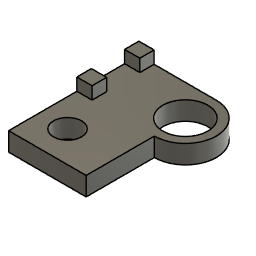
armservo v4 (Autodesk Fusion 360 design; units mm, degrees)
Autodesk Fusion 360 part; units mm, degrees
sketch "Esquisse1" plane through (0, 0, 0) normal (0, 1, 0) x (1, 0, 0)
  circle A0 centre (0, 0) radius 36.2394
  line L0 (-100, 50) -> (-125, 50)
  line L1 (-125, 50) -> (-125, -49.0109)
  circle A1 centre (0, 0) radius 50
  line L2 (-125, 50) -> (0, 50)
  line L3 (0, -50) -> (-125, -50)
  line L4 (-125, -50) -> (-125, 50)
  line L5 (-100, -50) -> (-100, -26.5854)
  line L6 (-100, -26.5854) -> (-124.9543, -26.5854)
  line L7 (-100, 50) -> (-100, 27)
  line L8 (-100, 27) -> (-125, 27)
  point P0 (-100, -50)
  point P1 (-100, -26.5854)
  point P2 (-100, 0)
  point P3 (-100, 27)
  point P4 (-100, 50)
  dimension "d3" = 100
  constraint horizontal L0
  constraint vertical L1
  constraint concentric A0 A1
  constraint horizontal L2
  constraint horizontal L3
  constraint vertical L4
  constraint coincident A1 L3.start
  constraint coincident L3 P0
  constraint coincident L0.start L7.start
  constraint coincident P0 L5.start
  constraint coincident P1 L5.end
  constraint perpendicular L3 L5
  constraint perpendicular L1 L6
  constraint coincident P4 L0.start
  constraint coincident P3 L7.end
  constraint perpendicular L2 L7
  constraint perpendicular L1 L8
  constraint coincident A1 L2.end
  constraint tangent A1 L2
  measures "d3" diameter of A1
extrude "Extrusion1" add sketch "Esquisse1" along normal blind 20 contours A1
sketch "Esquisse2" plane through (0, 20, 0) normal (0, 1, 0) x (-1, 0, 0)
  circle A0 centre (0, 0) radius 36.2394
  circle A1 centre (0, 0) radius 50
extrude "Extrusion3" add sketch "Esquisse1" along normal blind 20 contours L0 L1 L2 L4 L7 L8 | L1 A1 L2 L3 L4 L7 L8
sketch "Esquisse3" plane through (0, 20, 0) normal (0, 1, 0) x (-1, 0, 0)
  circle A0 centre (0, 0) radius 36.2394
  arc A1 (0, 50) -> (0, -50) centre (0, 0) ccw
  line L0 (0, -50) -> (125, -50)
  line L1 (125, -50) -> (125, 50)
  line L2 (125, 50) -> (0, 50)
  line L3 (125, -50) -> (100.4173, -50)
  line L4 (100.4173, -50) -> (100.4173, -26.9813)
  line L5 (100.4173, -26.9813) -> (125, -26.9813)
  line L6 (125, -26.9813) -> (125, -50)
  line L7 (125, 50) -> (100.4173, 50)
  line L8 (100.4173, 50) -> (100.4173, 26.5121)
  line L9 (100.4173, 26.5121) -> (125, 26.5121)
  line L10 (125, 26.5121) -> (125, 50)
  constraint horizontal L3
  constraint vertical L4
  constraint horizontal L5
  constraint vertical L6
  constraint coincident L0.end L1.start
  constraint horizontal L7
  constraint vertical L8
  constraint horizontal L9
  constraint vertical L10
  constraint coincident L1.end L2.start
extrude "Extrusion4" add sketch "Esquisse3" along normal blind 30 contours L1 L2 L7 L8 L9 L10 | L0 L1 L3 L4 L5 L6
sketch "Esquisse4" plane through (0, 0, 50) normal (0, 0, 1) x (1, 0, 0)
  line L0 (-125, 0) -> (0, 0)
  line L1 (0, 0) -> (0, 20)
  line L2 (0, 20) -> (-100.4173, 20)
  line L3 (-100.4173, 20) -> (-100.4173, 50)
  line L4 (-100.4173, 50) -> (-125, 50)
  line L5 (-125, 50) -> (-125, 0)
  line L6 (0, 0) -> (-125, 0)
  line L7 (-125, 0) -> (-125, 20)
  line L8 (-125, 20) -> (0, 20)
  line L9 (0, 20) -> (0, 0)
  constraint horizontal L6
  constraint vertical L7
  constraint horizontal L8
  constraint vertical L9
  constraint coincident L5 L7.end
  constraint coincident L0.end L1.start
extrude "Extrusion5" add sketch "Esquisse4" along normal blind 110 contours L0 L1 L2 L5 L6 L7 L8 L9
sketch "Esquisse5" plane through (0, 20, 0) normal (0, 1, 0) x (-1, 0, 0)
  line L0 (100.4173, 26.5121) -> (100.4173, 50)
  line L1 (100.4173, 50) -> (125, 50)
  line L2 (125, 50) -> (125, 160)
  line L3 (125, 160) -> (0, 160)
  line L4 (0, 160) -> (0, 50)
  arc A0 (0, 50) -> (0, -50) centre (0, 0) ccw
  line L5 (0, -50) -> (100.4173, -50)
  line L6 (100.4173, -50) -> (100.4173, -26.9813)
  line L7 (100.4173, -26.9813) -> (125, -26.9813)
  line L8 (125, -26.9813) -> (125, 26.5121)
  line L9 (125, 26.5121) -> (100.4173, 26.5121)
  circle A1 centre (0, 0) radius 36.2394
  circle A2 centre (80, 110) radius 25
  dimension "d14" = 50
  measures "d14" diameter of A2
extrude "Extrusion6" cut sketch "Esquisse5" against normal blind 20 contours A2
extrude "Extrusion7" cut 2 faces at (-108.6116, 50, -34.6542) (-108.6116, 50, 42.1707) along direction (0, -1, 0) blind 10
extrude "Extrusion8" add 1 faces at (-73.7992, 0, 13.676) along direction (0, -1, 0) blind 10
sketch "Esquisse6" plane through (0, 20, 0) normal (0, 1, 0) x (-1, 0, 0)
  circle A0 centre (80, 110) radius 25
  line L0 (100.4173, 26.5121) -> (100.4173, 50)
  line L1 (100.4173, 50) -> (125, 50)
  line L2 (125, 50) -> (125, 160)
  line L3 (125, 160) -> (0, 160)
  line L4 (0, 160) -> (0, 50)
  arc A1 (0, 50) -> (0, -50) centre (0, 0) ccw
  line L5 (0, -50) -> (100.4173, -50)
  line L6 (100.4173, -50) -> (100.4173, -26.9813)
  line L7 (100.4173, -26.9813) -> (125, -26.9813)
  line L8 (125, -26.9813) -> (125, 26.5121)
  line L9 (125, 26.5121) -> (100.4173, 26.5121)
  circle A2 centre (0, 0) radius 36.2394
  circle A3 centre (80, 110) radius 22.5
  dimension "d21" = 45
  constraint concentric A0 A3
  measures "d21" diameter of A3
move_face "DécalerLesFaces1" offset 2.5 1 faces at (-55.1242, 0, 112.4892)
extrude "Extrusion2" [suppressed]
